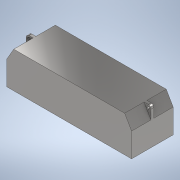
# Autodesk Inventor part: МПСТ Крышка корпуса
Saved by Autodesk Inventor 2022.1 (Build 261234020, 234B)
## iProperties
Created: 2021-11-18
Part Number: МПСТ Крышка корпуса
Material: Сталь, углеродистая
Document SubType Name: Modeling
Designer: Алексанян Г.
Density: 7.85 g/cm^3
Appearance: С умеренной полировкой
Author: Алексанян Г.
Autodesk Inventor part; units mm, degrees
ref_plane "YZ Plane" through (0, 0, 0) normal (1, 0, 0) x (0, 1, 0)
ref_plane "XZ Plane" through (0, 0, 0) normal (0, 1, 0) x (-1, 0, 0)
ref_plane "XY Plane" through (0, 0, 0) normal (0, 0, 1) x (1, 0, 0)
sketch "Эскиз1" plane through (0, 0, 0) normal (0, 1, 0) x (-1, 0, 0)
  line L0 (450, -150) -> (-450, -150)
  line L1 (-450, -150) -> (-450, 150)
  line L2 (-450, 150) -> (450, 150)
  line L3 (450, 150) -> (450, -150)
  line L4 (450, -150) -> (-450, 150) construction
  line L5 (-450, -150) -> (450, 150) construction
  point P0 (0, 0)
  dimension "d0" = 900
  dimension "d1" = 300
  constraints: 12 end point, 2 midpoint, 2 parallel, 1 horizontal, 1 perpendicular
  measures "d0" distance of L1.end L2.end
  measures "d1" distance of L0.end L1.end
extrude "Выдавливание1" add sketch "Эскиз1" along normal blind 260
sketch "Эскиз2" plane through (-450, 0, 150) normal (0, 0, 1) x (1, 0, 0)
  line L0 (0, 260) -> (900, 260) projected
  line L1 (50, 260) -> (0, 173.3975)
  line L2 (0, 0) -> (0, 260) projected
  line L3 (450, -56.4973) -> (450, 277.4189) construction
  line L4 (850, 260) -> (900, 173.3975)
  line L5 (0, 0) -> (900, 0) projected
  line L6 (900, 0) -> (900, 260) projected
  line L7 (900, 173.3975) -> (900, 260)
  point P0 (450, 0)
  point P1 (450, 0)
  dimension "d4" = 60
  dimension "d5" = 50
  constraints: 8 end point, 3 point on line, 2 symmetric about line, 2 vertical, 1 midpoint
  measures "d4" angle of L1 L0
  measures "d5" distance from line of L2 L1.start
extrude "Выдавливание2" cut sketch "Эскиз2" against normal through all contours L0 L1 L2 | L0 L6 L4
sketch "Эскиз3" plane through (0, 0, 0) normal (0, -1, 0) x (1, 0, 0)
  line L0 (-450, 150) -> (450, 150) projected
  point P0 (0, 0)
  point P1 (-228.7398, 140)
  dimension "d8" = 10
  measures "d8" distance from line of L0 point (-228.74, 140)
ref_plane "РабПлоскость1" through (-228.7398, 0, 140) normal (0, 0, 1) x (1, 0, 0)
sketch "Эскиз4" plane through (-228.7398, 0, 140) normal (0, 0, 1) x (1, 0, 0)
  line L0 (628.7398, 260) -> (678.7398, 173.3975) projected
  line L1 (678.7398, 0) -> (678.7398, 173.3975) projected
  line L2 (678.7398, 0) -> (-221.2602, 0) projected
  line L3 (-221.2602, 0) -> (-221.2602, 173.3975) projected
  line L4 (-221.2602, 173.3975) -> (-171.2602, 260) projected
  line L5 (628.7398, 260) -> (-171.2602, 260) projected
  line L6 (-165.4867, 250) -> (-211.2602, 170.718)
  line L7 (-211.2602, 170.718) -> (-211.2602, 0)
  line L8 (668.7398, 0) -> (668.7398, 170.718)
  line L9 (668.7398, 170.718) -> (622.9663, 250)
  line L10 (622.9663, 250) -> (-165.4867, 250)
  line L11 (-211.2602, 0) -> (668.7398, 0)
  line L12 (678.7398, 0) -> (-221.2602, 0) projected
  point P0 (228.7398, 0)
  dimension "d9" = 10
  dimension "d12" = 10
  constraints: 12 end point, 2 point on line, 1 collinear, 3 other
  measures "d9" distance between parallel lines of L5 L10
  measures "d12" distance between parallel lines of L3 L7
extrude "Выдавливание3" cut sketch "Эскиз4" against normal blind 280 contours L2 L7 L6 L10 L9 L8
sketch "Эскиз5" plane through (0, 0, 0) normal (0, 0, 1) x (1, 0, 0)
  line L0 (-400, 260) -> (-450, 260)
  line L1 (-450, 260) -> (-450, 173.3975)
  point P0 (0, 0)
  constraints: 4 end point, 1 horizontal, 1 perpendicular
extrude "Ребро жесткости1" add sketch "Эскиз5" along normal mid plane 20 rib yes fills toward (-425, 259.95) open curves L0 L1
fillet "Сопряжение1" radius 20 1 edges at (-450, 260, 0)
sketch "Эскиз6" plane through (-430, 260, 10) normal (0, 0, 1) x (1, 0, 0)
  arc A0 (0, 0) -> (-20, -20) centre (0, -20) ccw projected
  point P0 (430, -260)
  point P1 (0, -20)
  constraints: 1 coincident
hole "Отверстие1" at (-430, 240, 10) direction (0, 0, -1) diameter 20 end through all
mirror "Зеркальное отражение1" about plane through (0, 0, 0) normal (1, 0, 0) of "Ребро жесткости1", "Отверстие1"
fillet "Сопряжение2" radius 20 1 edges at (450, 260, 0)
